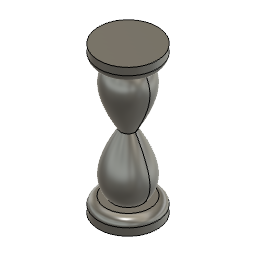
Hourglass (Autodesk Fusion 360 design; units mm, degrees)
part number: 2026-02-25-17-28-48-064
Autodesk Fusion 360 part; units mm, degrees
sketch "Sketch1" plane through (0, 0, 0) normal (0, 0, 1) x (1, 0, 0)
  line L0 (0, 0) -> (20, 0)
  line L1 (20, 0) -> (20, 10)
  line L2 (20, 10) -> (0, 10)
  line L3 (0, 10) -> (0, 50) construction
  line L4 (0, 10) -> (10, 10)
  line L5 (0, 10) -> (0, 23.3333) construction
  line L6 (0, 23.3333) -> (15, 23.3333) construction
  line L7 (0, 50) -> (5, 50) construction
  spline S0 degree 5 poles (10, 10) (10.4793, 10.5213) (11.3833, 11.5902) (12.5752, 13.2723) (13.8313, 15.6756) (14.8129, 18.9628) (15.1679, 22.5514) (14.8722, 26.4531) (13.9512, 30.6557) (12.4602, 35.1325) (10.4582, 39.8551) (8.4882, 43.8104) (6.8179, 46.8697) (5.62, 48.9498) (5, 50) knots 0 0 0 0 0 0 0.1 0.2 0.3 0.4 0.5 0.6 0.7 0.8 0.9 1 1 1 1 1 1
  line L8 (0, 10) -> (0, 13)
  line L9 (15, 23.3333) -> (12, 23.3333) construction
  line L10 (0, 13) -> (7, 13)
  line L11 (5, 50) -> (2, 50)
  spline S1 degree 5 poles (7, 13) (7.4867, 13.3807) (8.4033, 14.1767) (9.6085, 15.4748) (10.8699, 17.4172) (11.8386, 20.2177) (12.1643, 23.4119) (11.8344, 27.0077) (10.8883, 30.981) (9.3862, 35.2947) (7.3904, 39.9109) (5.4391, 43.8211) (3.7904, 46.8671) (2.6103, 48.9474) (2, 50) knots 0 0 0 0 0 0 0.1 0.2 0.3 0.4 0.5 0.6 0.7 0.8 0.9 1 1 1 1 1 1
  line L12 (0, 0) -> (0, 10)
  line L13 (0, 50) -> (5, 50) construction
  spline S2 degree 5 poles (7, 87) (7.4867, 86.6193) (8.4033, 85.8233) (9.6085, 84.5252) (10.8699, 82.5828) (11.8386, 79.7823) (12.1643, 76.5881) (11.8344, 72.9923) (10.8883, 69.019) (9.3862, 64.7053) (7.3904, 60.0891) (5.4391, 56.1789) (3.7904, 53.1329) (2.6103, 51.0526) (2, 50) knots 0 0 0 0 0 0 0.1 0.2 0.3 0.4 0.5 0.6 0.7 0.8 0.9 1 1 1 1 1 1
  line L14 (3.7291, 10.4414) -> (10.2709, 15.5586)
  line L15 (4.6467, 45.4353) -> (-0.6467, 54.5647)
  line L16 (3.7291, 89.5586) -> (10.2709, 84.4414)
  line L17 (4.6467, 54.5647) -> (-0.6467, 45.4353)
  line L18 (5, 50) -> (2, 50)
  line L19 (0, 90) -> (0, 76.6667) construction
  line L20 (15, 76.6667) -> (12, 76.6667) construction
  line L21 (0, 76.6667) -> (15, 76.6667) construction
  line L22 (0, 100) -> (0, 90)
  line L23 (20, 90) -> (0, 90)
  line L24 (0, 90) -> (0, 87)
  spline S3 degree 5 poles (10, 90) (10.4793, 89.4787) (11.3833, 88.4098) (12.5752, 86.7277) (13.8313, 84.3244) (14.8129, 81.0372) (15.1679, 77.4486) (14.8722, 73.5469) (13.9512, 69.3443) (12.4602, 64.8675) (10.4582, 60.1449) (8.4882, 56.1896) (6.8179, 53.1303) (5.62, 51.0502) (5, 50) knots 0 0 0 0 0 0 0.1 0.2 0.3 0.4 0.5 0.6 0.7 0.8 0.9 1 1 1 1 1 1
  line L25 (7.0166, 6.7552) -> (12.9834, 13.2448)
  line L26 (7.7565, 45.331) -> (2.2435, 54.669)
  line L27 (7.0166, 93.2448) -> (12.9834, 86.7552)
  line L28 (7.7565, 54.669) -> (2.2435, 45.331)
  line L29 (20, 100) -> (20, 90)
  line L30 (0, 90) -> (0, 50) construction
  line L31 (0, 87) -> (7, 87)
  line L32 (0, 90) -> (10, 90)
  line L33 (0, 100) -> (20, 100)
  point P0 (0, 100)
  dimension "d8" = 20
  dimension "d9" = 10
  dimension "d10" = 20
  dimension "d11" = 40
  dimension "d12" = 10
  dimension "d13" = 13.3333
  dimension "d14" = 15
  dimension "d15" = 5
  dimension "d17" = 3
  dimension "d18" = 3
  dimension "d19" = 7
  dimension "d20" = 3
  dimension "d21" = 10
  constraint coincident L0.start L12.start
  constraint horizontal L0
  constraint perpendicular L0 L1
  constraint perpendicular L1 L2
  constraint perpendicular L2 L3
  constraint perpendicular L3 L4
  constraint perpendicular L4 L5
  constraint perpendicular L5 L6
  constraint perpendicular L3 L7
  constraint perpendicular L4 L8
  constraint coincident L6.end L9.start
  constraint parallel L6 L9
  constraint perpendicular L8 L10
  constraint parallel L7 L11
  constraint perpendicular L2 L12
  constraint midpoint L10.end L14
  constraint midpoint L11.end L15
  constraint midpoint L4.end L25
  constraint midpoint L7.end L26
  constraint symmetric L0.start L7 L22.start
  constraint symmetric L0.start L7 P0
  constraint symmetric L0.end L7 L29.start
  constraint symmetric L1.end L7 L23.start
  constraint symmetric L2.end L7 L19.start
  constraint symmetric L3.end L7 L13.start
  constraint symmetric L4.end L7 S3.start
  constraint symmetric L5.end L7 L19.end
  constraint symmetric L6.end L7 L20.start
  constraint symmetric S0.end L7 L11.start
  constraint symmetric L7 L8.end L24.end
  constraint symmetric L7 L6.end L20.start
  constraint symmetric L7 L9.end L20.end
  constraint symmetric L7 L10.end S2.start
  constraint symmetric L7 L11.end S1.end
  constraint symmetric L7 L0.start P0
  constraint symmetric L7 L2.end L19.start
  constraint symmetric L7 L14.start L16.start
  constraint symmetric L7 L14.end L16.end
  constraint symmetric L7 L15.start L17.start
  constraint symmetric L7 L15.end L17.end
  constraint symmetric L7 L25.start L27.start
  constraint symmetric L7 L25.end L27.end
  constraint symmetric L7 L26.start L28.start
  constraint symmetric L7 L26.end L28.end
  measures "d8" distance of L0.start L0.end
  measures "d9" distance of L0.end L1.end
  measures "d10" distance of L1.end L2.end
  measures "d11" distance of L2.end L3.end
  measures "d12" distance of L2.end L4.end
  measures "d13" distance of L2.end L5.end
  measures "d14" distance of L5.end L6.end
  measures "d15" distance of L3.end L7.end
  measures "d17" distance of L2.end L8.end
  measures "d18" distance of L6.end L9.end
  measures "d19" distance of L8.end L10.end
  measures "d20" distance of L7.end L11.end
  measures "d21" distance of L0.start L2.end
revolve "Revolve1" add sketch "Sketch1" angle 360 about axis through (0, 90, 0) along (0, -1, 0)
fillet "Fillet1" radius 5 2 edges at (-18.6465, 90, -7.2323) (-18.6465, 10, -7.2323)
equation "base_d = 40 mm"
equation "base_thick = 10 mm"
equation "half_height = 40 mm"
equation "widest_d = 30 mm"
equation "end_d = 20 mm"
equation "center_d = 10 mm"
equation "glass_thick = 3 mm"
equation "d8 = base_d / 2"
equation "d9 = base_thick"
equation "d10 = base_d / 2"
equation "d11 = half_height"
equation "d12 = end_d / 2"
equation "d13 = half_height / 3"
equation "d14 = widest_d / 2"
equation "d15 = center_d / 2"
equation "d17 = glass_thick"
equation "d18 = glass_thick"
equation "d19 = ( end_d / 2 ) - glass_thick"
equation "d20 = glass_thick"
equation "d21 = base_thick"
